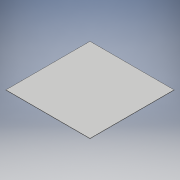
# Autodesk Inventor part: Pit Station floor
Saved by Autodesk Inventor 2019.4 (Build 234330000, 330)
## iProperties
Created: 2020-02-27
Part Number: Pit Station floor
Material: Generic
Document SubType Name: Modeling
Designer: admin
Density: 1 g/cm^3
Appearance: Default
Author: admin
Autodesk Inventor part; units mm, degrees
ref_plane "YZ Plane" through (0, 0, 0) normal (1, 0, 0) x (0, 1, 0)
ref_plane "XZ Plane" through (0, 0, 0) normal (0, 1, 0) x (-1, 0, 0)
ref_plane "XY Plane" through (0, 0, 0) normal (0, 0, 1) x (1, 0, 0)
sketch "Sketch1" plane through (0, 0, 0) normal (0, 1, 0) x (-1, 0, 0)
  line L0 (-1500, 1500) -> (1500, 1500)
  line L1 (1500, 1500) -> (1500, -1500)
  line L2 (1500, -1500) -> (-1500, -1500)
  line L3 (-1500, -1500) -> (-1500, 1500)
  line L4 (-1500, 1500) -> (1500, -1500) construction
  line L5 (1500, 1500) -> (-1500, -1500) construction
  point P0 (0, 0)
  dimension "d0" = 3000
  dimension "d1" = 3000
  constraints: 12 end point, 2 midpoint, 2 parallel, 1 horizontal, 1 perpendicular
  measures "d0" distance of L1.end L2.end
  measures "d1" distance of L0.end L1.end
extrude "Extrusion1" add sketch "Sketch1" along normal blind 10
body "Solid1"
